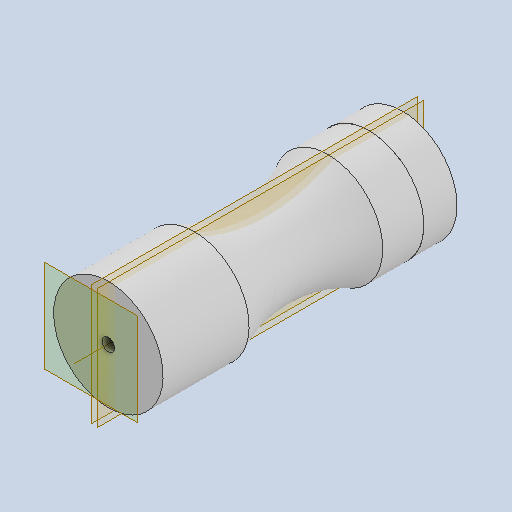
# Autodesk Inventor part: Roller_Drib_v2
Saved by Autodesk Inventor 2025.1 (Build 291241000, 241)
## iProperties
Created: 2026-05-05
Part Number: Roller_Drib_v2
Material: Generic
Document SubType Name: Modeling
Designer: User
Density: 1 g/cm^3
Appearance: Default
Author: User
## iProperties of the stored document Roller_Drib_v2_3DPrint.ipt
Created: 2026-05-06
Part Number: Roller_Drib_v2_3DPrint
Material: Generic
Document SubType Name: Modeling
Designer: User
Density: 1 g/cm^3
Appearance: Default
Author: User
Autodesk Inventor part; units mm, degrees
ref_plane "YZ Plane" through (0, 0, 0) normal (1, 0, 0) x (0, 1, 0)
ref_plane "XZ Plane" through (0, 0, 0) normal (0, 1, 0) x (-1, 0, 0)
ref_plane "XY Plane" through (0, 0, 0) normal (0, 0, 1) x (1, 0, 0)
sketch "Sketch1" plane through (0, 0, 0) normal (0, 0, 1) x (1, 0, 0)
  spline S0 degree 3 poles (1.875, 3.375) (2.0588, 3.375) (2.2411, 3.3412) (2.5681, 3.2156) (2.7123, 3.1306) (2.993, 2.8949) (3.119, 2.7368) (3.2515, 2.478) (3.2853, 2.3938) (3.3675, 2.1205) (3.3868, 1.9249) (3.3551, 1.597) (3.3243, 1.4655) (3.2519, 1.2759) (3.2231, 1.2138) (3.0962, 0.9823) (2.9695, 0.8308) (2.6755, 0.5935) (2.5143, 0.5059) (2.1978, 0.4024) (2.0482, 0.3774) (1.8146, 0.3739) (1.7319, 0.3796) (1.5112, 0.413) (1.3761, 0.4535) (1.1124, 0.5746) (0.9866, 0.6572) (0.875, 0.757) knots -0.582189 -0.582189 -0.582189 -0.582189 -0.527 -0.527 -0.477091 -0.477091 -0.416978 -0.416978 -0.389781 -0.389781 -0.331291 -0.331291 -0.290926 -0.290926 -0.270407 -0.270407 -0.211701 -0.211701 -0.157129 -0.157129 -0.11191 -0.11191 -0.087075 -0.087075 -0.044972 -0.044972 -0.000067 -0.000067 -0.000067 -0.000067 projected
  arc A0 (1.875, 3.375) -> (0.8751, 2.9931) centre (1.875, 1.875) ccw projected
  line L0 (0.875, 2.7063) -> (0.875, 2.9933) projected
  line L1 (0.875, 0.757) -> (0.875, 1.0434) projected
  line L2 (0.875, 1.0434) -> (0.875, 2.7063) projected
  arc A1 (1.875, 3.375) -> (0.8751, 2.9931) centre (1.875, 1.875) ccw projected
  arc A2 (1.875, 3.375) -> (0.8751, 2.9931) centre (1.875, 1.875) ccw projected
  line L3 (0.875, 2.7063) -> (0.875, 2.9933) projected
  arc A3 (1.875, 3.375) -> (0.8751, 2.9931) centre (1.875, 1.875) ccw projected
  line L4 (0.8751, 2.9931) -> (0.875, 2.993)
  arc A4 (1.875, 3.475) -> (0.8084, 3.0676) centre (1.875, 1.875) ccw
  line L5 (0.775, 2.7063) -> (0.775, 1.0434)
  line L6 (0.775, 1.0434) -> (0.775, 0.757)
  arc A5 (0.775, 0.7131) -> (0.775, 3.0369) centre (1.875, 1.875) ccw
  line L7 (0.775, 0.7131) -> (0.775, 3.0369)
  line L8 (-1.225, 3.7053) -> (-1.225, 0.0447)
  arc A6 (-1.225, 0.0447) -> (-1.225, 3.7053) centre (1.875, 1.875) ccw
  spline S1 degree 5 poles (1.875, 3.475) (2.4931, 3.4741) (3.1161, 3.179) (3.5324, 2.5696) (3.6487, 1.1994) (2.6504, 0.2531) (1.9326, 0.0751) (1.2703, 0.2704) (0.8083, 0.6824) knots 0 0 0 0 0 0 0.499643 0.499643 0.499643 1 1 1 1 1 1
  point P0 (0, 0)
  point P1 (0.8084, 3.0676)
  dimension "d0" = 0.1
  dimension "d1" = 0.1
  dimension "d2" = 0.1
  dimension "d3" = 2
  constraints: 10 end point, 8 point on circle, 3 centre point, 3 point on line, 1 coincident, 5 other
  measures "d1" radial gap between concentric circles of A0 A4
  measures "d2" distance between parallel lines of L2 L5
  measures "d3" radial gap between concentric circles of A5 A6
extrude "Extrusion1" add sketch "Sketch1" against normal blind 7.5 contours A6 L8
sketch "Sketch2" plane through (0, 0, -7.5) normal (0, 0, -1) x (-1, 0, 0)
  arc A0 (-0.775, 3.0369) -> (-0.775, 0.7131) centre (-1.875, 1.875) ccw projected
  line L0 (11.7103, -4.6309) -> (11.7078, 0.3691) projected
  line L1 (11.7078, 0.3691) -> (11.7078, 0.3708) projected
  line L2 (11.7078, 0.3708) -> (11.7103, -4.6291) projected
  line L3 (11.7103, -4.6291) -> (11.7103, -4.6309) projected
  circle A1 centre (-1.875, 1.875) radius 13
  line L4 (-0.775, 3.0369) -> (-0.775, 0.7131) projected
  point P0 (0, 0)
  dimension "d6" = 26
  constraints: 1 centre point, 1 coincident
  measures "d6" diameter of A1
extrude "Extrusion2" add sketch "Sketch2" against normal blind 7.5
ref_plane "Work Plane2" through (4.7942, 7.2328, 69.481) normal (0, 0, -1) x (-1, 0, 0)
ref_plane "Work Plane5" through (1.975, 1.8749, 0) normal (0.9999999, -0.0005003, 0.0000004) x (0.0005003, 0.9999999, -0.0000344)
ref_plane "Work Plane4" through (3.475, 1.8742, 0) normal (0.9999999, -0.0005003, 0.0000004) x (0.0005003, 0.9999999, -0.0000344)
sketch "Sketch4" plane through (1.975, 1.8749, 0) normal (0.9999999, -0.0005003, 0.0000004) x (0.0005003, 0.9999999, -0.0000344)
  arc A0 (-12.9997, 10.2701) -> (-12.9997, 42.0339) centre (-44.1889, 26.152) ccw
  line L0 (-12.9997, -7.5004) -> (-13, -0.0004) projected
  line L1 (0, 62.4812) -> (-12.9997, 62.4812)
  line L2 (-12.9997, 62.4812) -> (-12.9997, 42.0339)
  ellipse E0 centre (0, 0) end of major axis (-13, -0.0004) minor radius 0 projected
  ellipse E1 centre (0.0003, -7.5) end of major axis (13.0003, -7.4996) minor radius 0 projected
  line L3 (0, 0) -> (-12.9997, 0)
  line L4 (-12.9997, 0.4906) -> (0, 0.4906)
  line L5 (-12.9997, 0.4906) -> (0, 0.4906) construction
  line L6 (0, 0.4906) -> (0, 62.4812)
  line L7 (-12.9997, -0.0004) -> (-12.9997, 0)
  line L8 (-12.9997, 0.4906) -> (-12.9997, 10.2701)
  point P0 (0, 0.4906)
  constraints: 16 end point, 3 perpendicular, 2 point on circle, 1 centre point, 1 collinear, 1 horizontal, 1 vertical, 4 other
revolve "Revolution1" add sketch "Sketch4" angle 360 about axis through (1.975, 1.875, 0.4906) along (-0.0000004, 0.0000344, 1)
sketch "Sketch5" plane through (1.875, 1.875, 0) normal (0, 0, 1) x (1, 0, 0)
  circle A0 centre (0, 0) radius 13 projected
  line L0 (-1.1, -1.1619) -> (-1.1, 1.1619) projected
  arc A1 (-1.1, -1.1619) -> (-1.1, 1.1619) centre (0, 0) ccw projected
  point P0 (-1.875, -1.875)
extrude "Extrusion3" add sketch "Sketch5" along normal up to surface (0.4906 mm away)
sketch "Sketch6" plane through (1.975, 1.8771, 62.4812) normal (-0.0000004, 0.0000344, 1) x (1, 0, 0.0000004)
  circle A0 centre (0, 0) radius 12.9997 projected
  circle A1 centre (0, 0) radius 1.5
  point P0 (-1.975, -1.8749)
  dimension "d18" = 3
  constraints: 1 centre point, 1 coincident
  measures "d18" diameter of A1
extrude "Extrusion4" cut sketch "Sketch6" against normal blind 16 contours A1
ref_plane "Work Plane3" through (7.9717, -4.6381, 64.4814) normal (0.9999999, -0.0005003, 0.0000004) x (0.0005003, 0.9999999, -0.0000344)
body "Solid1"
